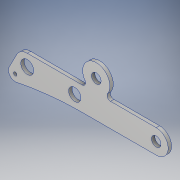
# Autodesk Inventor part: Intake Arm
Saved by Autodesk Inventor 2019.4 (Build 234330000, 330)
## iProperties
Created: 2020-01-28
Part Number: Intake Arm
Material: Aluminum 6061
Document SubType Name: Modeling
Designer: admin
Density: 2.7 g/cm^3
Appearance: Aluminum - Flat
Mass: 104.947 g
Surface Area: 187.284 cm^2
Volume: 38.8691 cm^3
Author: admin
Autodesk Inventor part; units mm, degrees
ref_plane "YZ Plane" through (0, 0, 0) normal (1, 0, 0) x (0, 1, 0)
ref_plane "XZ Plane" through (0, 0, 0) normal (0, 1, 0) x (-1, 0, 0)
ref_plane "XY Plane" through (0, 0, 0) normal (0, 0, 1) x (1, 0, 0)
sketch "Sketch1" plane through (0, 0, 0) normal (0, 0, 1) x (1, 0, 0)
  circle A0 centre (0, 0) radius 9.5
  arc A1 (0, -17.5) -> (0, 17.5) centre (0, 0) ccw construction
  circle A2 centre (190, 0) radius 7
  circle A3 centre (-175.4753, -121.2237) radius 88.9 construction
  circle A4 centre (190, 0) radius 41.275 construction
  circle A5 centre (190, 0) radius 28.5 construction
  line L0 (-263.1536, 888.7662) -> (-263.1536, -773.9924) construction
  line L1 (0, 0) -> (190, 0) construction
  arc A6 (190, 17.5) -> (190, -17.5) centre (190, 0) ccw construction
  line L2 (190, 17.5) -> (108.4742, 17.5)
  line L3 (190, -17.5) -> (0, -17.5)
  arc A7 (0, 17.5) -> (-15.5167, 8.0921) centre (0, 0) ccw
  arc A8 (190, -17.5) -> (190, 17.5) centre (190, 0) ccw
  line L4 (0, 0) -> (263.9458, 0) construction
  circle A9 centre (-17.6777, -17.6777) radius 2.5
  circle A10 centre (-17.6777, -17.6777) radius 10
  line L5 (-17.6777, -17.6777) -> (0, 0) construction
  circle A11 centre (-30, 150) radius 2.5 construction
  line L6 (-30, 150) -> (-17.6777, -17.6777) construction
  line L7 (0, -17.5) -> (-11.9385, -25.8668)
  line L8 (-26.5444, -13.0536) -> (-15.5167, 8.0921)
  arc A12 (-15.5167, 8.0921) -> (0, -17.5) centre (0, 0) ccw construction
  line L9 (190, 0) -> (101.6671, 36.3059) construction
  circle A13 centre (70, 0) radius 9
  circle A14 centre (101.6671, 36.3059) radius 7
  line L10 (70, 0) -> (101.6671, 36.3059) construction
  arc A15 (108.4742, 17.5) -> (94.86, 17.5) centre (101.6671, 36.3059) ccw
  arc A16 (94.86, 17.5) -> (108.4742, 17.5) centre (101.6671, 36.3059) ccw construction
  line L11 (94.86, 17.5) -> (0, 17.5)
  line L12 (108.4742, 17.5) -> (94.86, 17.5) construction
  dimension "d0" = 19
  dimension "d1" = 35
  dimension "d4" = 14
  dimension "d5" = 177.8
  dimension "d6" = 82.55
  dimension "d7" = 57
  dimension "d8" = 190
  dimension "d9" = 35
  dimension "d10" = 0
  dimension "d11" = 5
  dimension "d12" = 20
  dimension "d13" = 25
  dimension "d14" = 135
  dimension "d15" = 5
  dimension "d16" = 150
  dimension "d17" = 30
  dimension "d18" = 168.1298
  dimension "d20" = 95.503
  dimension "d21" = 18
  dimension "d22" = 14
  dimension "d23" = 48.176
  dimension "d24" = 40
  dimension "d25" = 70
  constraints: 26 end point, 17 centre point, 16 point on circle, 12 tangent, 8 coincident, 1 horizontal, 1 point on line, 1 vertical
  measures "d0" diameter of A0
  measures "d1" diameter of A1
  measures "d4" diameter of A2
  measures "d5" diameter of A3
  measures "d6" diameter of A4
  measures "d7" diameter of A5
  measures "d8" distance of L1.start L1.end
  measures "d9" diameter of A6
  measures "d10" distance between parallel lines of L1 L4
  measures "d11" diameter of A9
  measures "d12" diameter of A10
  measures "d13" distance of L5.start L1.start
  measures "d14" angle of L1 L5
  measures "d15" diameter of A11
  measures "d16" vertical distance of A0.centre L6.start
  measures "d17" horizontal distance of A0.centre L6.start
  measures "d18" distance of L6.start L5.start
  measures "d20" distance of L9.start L9.end
  measures "d21" diameter of A13
  measures "d22" diameter of A14
  measures "d23" distance of L10.start L10.end
  measures "d24" diameter of A15
  measures "d25" distance of point (0, 0) L10.start
extrude "Extrusion1" add sketch "Sketch1" along normal blind 5
fillet "Fillet1" radius 500 1 edges at (0, -17.5, 2.5)
fillet "Fillet2" radius 5 2 edges at (108.4742, 17.5, 2.5) (94.86, 17.5, 2.5)
body "Solid1"
